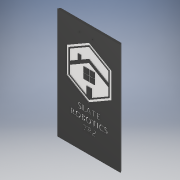
# Autodesk Inventor part: BA03
Saved by Autodesk Inventor 2017 (Build 210142000, 142)
## iProperties
Created: 2018-10-18
Part Number: BA03
Material: ABS Plastic
Document SubType Name: Modeling
Designer: Dell
Density: 1.06 g/cm^3
Appearance: Smooth - Black
Author: Dell
Autodesk Inventor part; units mm, degrees
ref_plane "YZ Plane" through (0, 0, 0) normal (1, 0, 0) x (0, 1, 0)
ref_plane "XZ Plane" through (0, 0, 0) normal (0, 1, 0) x (-1, 0, 0)
ref_plane "XY Plane" through (0, 0, 0) normal (0, 0, 1) x (1, 0, 0)
sketch "Sketch1" plane through (0, 0, 0) normal (0, 0, 1) x (1, 0, 0)
  line L0 (0, 0) -> (292.1, 0)
  line L1 (292.1, 0) -> (292.1, -533.4)
  line L2 (292.1, -533.4) -> (0, -533.4)
  line L3 (0, -533.4) -> (0, 0)
  dimension "d0" = 292.1
  dimension "d1" = 533.4
  constraints: 8 end point, 2 parallel, 1 horizontal, 1 perpendicular
  measures "d0" distance of L1.end L2.end
  measures "d1" distance of L0.end L1.end
extrude "Extrusion1" add sketch "Sketch1" along normal blind 10
sketch "Sketch2" plane through (0, 0, 0) normal (0, 1, 0) x (1, 0, 0)
  line L0 (292.1, -10) -> (0, -10) projected
  line L1 (0, -10) -> (-5.7735, -10)
  line L2 (-5.7735, -10) -> (0, 0)
  line L3 (0, 0) -> (0, -10) projected
  line L4 (0, 0) -> (0, -10) projected
  line L5 (0, -10) -> (0, 0)
  line L6 (292.1, -10) -> (297.8735, -10)
  line L7 (292.1, 0) -> (292.1, -10) projected
  line L8 (297.8735, -10) -> (292.1, 0)
  line L9 (292.1, 0) -> (292.1, -10)
  dimension "d4" = 30
  dimension "d5" = 60
  constraints: 12 end point, 2 collinear, 2 horizontal
  measures "d4" angle of L3 L2
  measures "d5" angle of L6 L8
extrude "Extrusion2" add sketch "Sketch2" against normal blind 533.4
sketch "Sketch5" plane through (0, 0, 10) normal (0, 0, 1) x (1, 0, 0)
  circle A0 centre (101, -44.45) radius 2.3812
  circle A1 centre (164.5, -44.45) radius 2.3813
  line L0 (-5.7735, 0) -> (297.8735, 0) projected
  line L1 (-5.7735, 0) -> (-5.7735, -533.4) projected
  line L2 (0, -533.4) -> (0, 0) projected
  dimension "d18" = 4.7625
  dimension "d19" = 63.5
  dimension "d20" = 4.7625
  dimension "d21" = 44.45
  dimension "d23" = 101
  constraints: 2 centre point, 1 horizontal alignment
  measures "d18" diameter of A0
  measures "d19" distance of A0.centre A1.centre
  measures "d20" diameter of A1
  measures "d21" distance from line of L0 A0.centre
  measures "d23" distance from line of A0.centre L2
extrude "Extrusion4" cut sketch "Sketch5" against normal through all
sketch "Sketch6" plane through (0, 0, 10) normal (0, 0, 1) x (1, 0, 0)
  line L0 (21.05, -316.7) -> (271.05, -316.7) construction
  line L1 (271.05, -316.7) -> (271.05, -466.7) construction
  line L2 (271.05, -466.7) -> (21.05, -466.7) construction
  line L3 (21.05, -466.7) -> (21.05, -316.7) construction
  line L4 (21.05, -66.7) -> (271.05, -66.7) construction
  line L5 (271.05, -66.7) -> (271.05, -316.7) construction
  line L6 (271.05, -316.7) -> (21.05, -316.7) construction
  line L7 (21.05, -316.7) -> (21.05, -66.7) construction
  line L8 (271.05, -466.7) -> (271.05, -66.7) construction
  line L9 (146.05, -66.7) -> (254.3032, -129.2)
  line L10 (254.3032, -129.2) -> (254.3032, -254.2)
  line L11 (254.3032, -254.2) -> (146.05, -316.7)
  line L12 (146.05, -316.7) -> (37.7968, -254.2)
  line L13 (37.7968, -254.2) -> (37.7968, -129.2)
  line L14 (37.7968, -129.2) -> (146.05, -66.7)
  line L15 (146.05, -78.4779) -> (244.1032, -135.089)
  line L16 (244.1032, -135.089) -> (244.1032, -248.311)
  line L17 (244.1032, -248.311) -> (146.05, -304.9221)
  line L18 (146.05, -304.9221) -> (47.9968, -248.311)
  line L19 (47.9968, -248.311) -> (47.9968, -135.089)
  line L20 (47.9968, -135.089) -> (146.05, -78.4779)
  line L21 (146.05, -83.3854) -> (239.8532, -137.5427) construction
  line L22 (239.8532, -137.5427) -> (239.8532, -245.8573) construction
  line L23 (239.8532, -245.8573) -> (146.05, -300.0146) construction
  line L24 (146.05, -300.0146) -> (52.2468, -245.8573) construction
  line L25 (52.2468, -245.8573) -> (52.2468, -137.5427) construction
  line L26 (52.2468, -137.5427) -> (146.05, -83.3854) construction
  line L27 (52.2468, -190.0427) -> (92.2468, -166.9487)
  line L28 (92.2468, -166.9487) -> (92.2468, -138.4487)
  line L29 (92.2468, -138.4487) -> (106.2468, -138.4487)
  line L30 (106.2468, -138.4487) -> (106.2468, -158.8658)
  line L31 (106.2468, -158.8658) -> (146.05, -135.8854)
  line L32 (146.05, -135.8854) -> (239.8532, -190.0427)
  line L33 (239.8532, -190.0427) -> (239.8532, -137.5427)
  line L34 (239.8532, -137.5427) -> (146.05, -83.3854)
  line L35 (146.05, -83.3854) -> (52.2468, -137.5427)
  line L36 (52.2468, -190.0427) -> (52.2468, -137.5427)
  line L37 (52.2468, -245.8573) -> (134.05, -293.0864)
  line L38 (134.05, -293.0864) -> (134.05, -253.0146)
  line L39 (134.05, -253.0146) -> (158.05, -253.0146)
  line L40 (158.05, -253.0146) -> (158.05, -293.0864)
  line L41 (158.05, -293.0864) -> (239.8532, -245.8573)
  line L42 (239.8532, -245.8573) -> (239.8532, -205.0427)
  line L43 (239.8532, -205.0427) -> (146.05, -150.8854)
  line L44 (146.05, -150.8854) -> (52.2468, -205.0427)
  line L45 (52.2468, -205.0427) -> (52.2468, -245.8573)
  line L46 (119.8, -179.0146) -> (172.3, -179.0146) construction
  line L47 (172.3, -179.0146) -> (172.3, -230.0146) construction
  line L48 (172.3, -230.0146) -> (119.8, -230.0146) construction
  line L49 (119.8, -230.0146) -> (119.8, -179.0146) construction
  line L50 (119.8, -230.0146) -> (143.8, -230.0146)
  line L51 (143.8, -230.0146) -> (143.8, -206.0146)
  line L52 (143.8, -206.0146) -> (119.8, -206.0146)
  line L53 (119.8, -206.0146) -> (119.8, -230.0146)
  line L54 (119.8, -179.0146) -> (143.8, -179.0146)
  line L55 (143.8, -179.0146) -> (143.8, -203.0146)
  line L56 (143.8, -203.0146) -> (119.8, -203.0146)
  line L57 (119.8, -203.0146) -> (119.8, -179.0146)
  line L58 (172.3, -179.0146) -> (148.3, -179.0146)
  line L59 (148.3, -179.0146) -> (148.3, -203.0146)
  line L60 (148.3, -203.0146) -> (172.3, -203.0146)
  line L61 (172.3, -203.0146) -> (172.3, -179.0146)
  line L62 (172.3, -230.0146) -> (148.3, -230.0146)
  line L63 (148.3, -230.0146) -> (148.3, -206.0146)
  line L64 (148.3, -206.0146) -> (172.3, -206.0146)
  line L65 (172.3, -206.0146) -> (172.3, -230.0146)
  line L66 (-5.7735, 0) -> (297.8735, 0) projected
  line L67 (-5.7735, 0) -> (-5.7735, -533.4) projected
  line L68 (92.7983, -364.3042) -> (92.7983, -360.0196)
  spline S0 degree 2 poles (92.7983, -360.0196) (95.7248, -361.2437) (98.6131, -361.7219) (99.8182, -361.7219) knots 0 0 0 1 2 2 2
  spline S1 degree 2 poles (99.8182, -361.7219) (101.9987, -361.7219) (104.1602, -359.7709) (104.1602, -358.3937) knots 0 0 0 1 2 2 2
  spline S2 degree 2 poles (104.1602, -358.3937) (104.1602, -357.3417) (103.5672, -356.5) knots 0 0 0 1 1 1
  spline S3 degree 2 poles (103.5672, -356.5) (102.9551, -355.6776) (100.6024, -354.3577) knots 0 0 0 1 1 1
  line L69 (100.6024, -354.3577) -> (98.9192, -353.4205)
  spline S4 degree 2 poles (98.9192, -353.4205) (95.304, -351.4121) (94.0416, -349.7097) knots 0 0 0 1 1 1
  spline S5 degree 2 poles (94.0416, -349.7097) (92.7409, -348.0073) (92.7409, -345.7694) knots 0 0 0 1 1 1
  spline S6 degree 2 poles (92.7409, -345.7694) (92.7409, -342.9385) (97.0638, -338.9216) (101.0997, -338.9216) knots 0 0 0 1 2 2 2
  spline S7 degree 2 poles (101.0997, -338.9216) (104.1219, -338.9216) (107.9092, -339.7824) knots 0 0 0 1 1 1
  line L70 (107.9092, -339.7824) -> (107.9092, -343.7801)
  spline S8 degree 2 poles (107.9092, -343.7801) (104.0263, -342.3455) (101.7501, -342.3455) knots 0 0 0 1 1 1
  spline S9 degree 2 poles (101.7501, -342.3455) (99.8564, -342.3455) (97.8863, -343.9905) (97.8863, -345.1382) knots 0 0 0 1 2 2 2
  spline S10 degree 2 poles (97.8863, -345.1382) (97.8863, -346.018) (98.4984, -346.764) knots 0 0 0 1 1 1
  spline S11 degree 2 poles (98.4984, -346.764) (99.0722, -347.5291) (101.4249, -348.8489) knots 0 0 0 1 1 1
  line L71 (101.4249, -348.8489) -> (103.2229, -349.8436)
  spline S12 degree 2 poles (103.2229, -349.8436) (107.3736, -352.158) (108.5022, -353.8604) knots 0 0 0 1 1 1
  spline S13 degree 2 poles (108.5022, -353.8604) (109.6307, -355.5819) (109.6307, -357.7242) knots 0 0 0 1 1 1
  spline S14 degree 2 poles (109.6307, -357.7242) (109.6307, -360.8038) (104.9444, -365.1458) (99.8373, -365.1458) knots 0 0 0 1 2 2 2
  spline S15 degree 2 poles (99.8373, -365.1458) (96.8151, -365.1458) (92.7983, -364.3042) knots 0 0 0 1 1 1
  line L72 (113.9536, -364.5337) -> (113.9536, -339.5337)
  line L73 (113.9536, -339.5337) -> (119.1564, -339.5337)
  line L74 (119.1564, -339.5337) -> (119.1564, -360.9951)
  line L75 (119.1564, -360.9951) -> (130.3078, -360.9951)
  line L76 (130.3078, -360.9951) -> (130.3078, -364.5337)
  line L77 (130.3078, -364.5337) -> (113.9536, -364.5337)
  line L78 (131.3216, -364.5337) -> (141.0194, -339.5337)
  line L79 (141.0194, -339.5337) -> (146.2413, -339.5337)
  line L80 (146.2413, -339.5337) -> (155.9773, -364.5337)
  line L81 (155.9773, -364.5337) -> (150.6407, -364.5337)
  line L82 (150.6407, -364.5337) -> (148.0393, -357.8581)
  line L83 (148.0393, -357.8581) -> (137.7103, -357.8581)
  line L84 (137.7103, -357.8581) -> (135.1089, -364.5337)
  line L85 (135.1089, -364.5337) -> (131.3216, -364.5337)
  line L86 (138.9919, -354.5299) -> (146.7386, -354.5299)
  line L87 (146.7386, -354.5299) -> (142.8748, -344.5643)
  line L88 (142.8748, -344.5643) -> (138.9919, -354.5299)
  line L89 (165.7325, -364.5337) -> (165.7325, -342.9767)
  line L90 (165.7325, -342.9767) -> (156.7807, -342.9767)
  line L91 (156.7807, -342.9767) -> (156.7807, -339.5337)
  line L92 (156.7807, -339.5337) -> (179.887, -339.5337)
  line L93 (179.887, -339.5337) -> (179.887, -342.9767)
  line L94 (179.887, -342.9767) -> (170.9352, -342.9767)
  line L95 (170.9352, -342.9767) -> (170.9352, -364.5337)
  line L96 (170.9352, -364.5337) -> (165.7325, -364.5337)
  line L97 (183.3683, -364.5337) -> (183.3683, -339.5337)
  line L98 (183.3683, -339.5337) -> (199.3782, -339.5337)
  line L99 (199.3782, -339.5337) -> (199.3782, -342.9767)
  line L100 (199.3782, -342.9767) -> (188.571, -342.9767)
  line L101 (188.571, -342.9767) -> (188.571, -349.9392)
  line L102 (188.571, -349.9392) -> (197.5037, -349.9392)
  line L103 (197.5037, -349.9392) -> (197.5037, -353.3822)
  line L104 (197.5037, -353.3822) -> (188.571, -353.3822)
  line L105 (188.571, -353.3822) -> (188.571, -360.9951)
  line L106 (188.571, -360.9951) -> (200.1816, -360.9951)
  line L107 (200.1816, -360.9951) -> (200.1816, -364.5337)
  line L108 (200.1816, -364.5337) -> (183.3683, -364.5337)
  line L109 (58.0336, -404.4902) -> (58.0336, -379.4902)
  line L110 (58.0336, -379.4902) -> (67.387, -379.4902)
  spline S16 degree 2 poles (67.387, -379.4902) (70.2562, -379.4902) (73.2593, -380.9248) (74.9999, -383.8514) (74.9999, -385.6876) knots 0 0 0 1 2 3 3 3
  spline S17 degree 2 poles (74.9999, -385.6876) (74.9999, -387.8873) (72.475, -391.7894) (70.1606, -392.8223) knots 0 0 0 1 2 2 2
  line L111 (70.1606, -392.8223) -> (78.3281, -404.4902)
  line L112 (78.3281, -404.4902) -> (71.9968, -404.4902)
  line L113 (71.9968, -404.4902) -> (65.7803, -394.276)
  line L114 (65.7803, -394.276) -> (62.9303, -394.276)
  line L115 (62.9303, -394.276) -> (62.9303, -404.4902)
  line L116 (62.9303, -404.4902) -> (58.0336, -404.4902)
  line L117 (62.9303, -390.8521) -> (64.1162, -390.8521)
  spline S18 degree 2 poles (64.1162, -390.8521) (67.3297, -390.8521) (69.7971, -388.0403) (69.7971, -386.2615) knots 0 0 0 1 2 2 2
  spline S19 degree 2 poles (69.7971, -386.2615) (69.7971, -384.7312) (67.8078, -382.9141) (64.7474, -382.9141) knots 0 0 0 1 2 2 2
  line L118 (64.7474, -382.9141) -> (62.9303, -382.9141)
  line L119 (62.9303, -382.9141) -> (62.9303, -390.8521)
  spline S20 degree 2 poles (93.0183, -405.1023) (89.1162, -405.1023) (83.3396, -401.8697) (80.3365, -395.8253) (80.3365, -391.9807) knots 0 0 0 1 2 3 3 3
  spline S21 degree 2 poles (80.3365, -391.9807) (80.3365, -388.1742) (83.3396, -382.0916) (89.1544, -378.8781) (93.0183, -378.8781) knots 0 0 0 1 2 3 3 3
  spline S22 degree 2 poles (93.0183, -378.8781) (96.8629, -378.8781) (102.6778, -382.0916) (105.6808, -388.1742) (105.6808, -391.9807) knots 0 0 0 1 2 3 3 3
  spline S23 degree 2 poles (105.6808, -391.9807) (105.6808, -395.8253) (102.6778, -401.8697) (96.9203, -405.1023) (93.0183, -405.1023) knots 0 0 0 1 2 3 3 3
  spline S24 degree 2 poles (93.0183, -401.6784) (96.6334, -401.6784) (100.1529, -395.7871) (100.1529, -391.9807) knots 0 0 0 1 2 2 2
  spline S25 degree 2 poles (100.1529, -391.9807) (100.1529, -388.1551) (96.6143, -382.302) (93.0183, -382.302) knots 0 0 0 1 2 2 2
  spline S26 degree 2 poles (93.0183, -382.302) (89.4031, -382.302) (85.8645, -388.1551) (85.8645, -391.9807) knots 0 0 0 1 2 2 2
  spline S27 degree 2 poles (85.8645, -391.9807) (85.8645, -395.7871) (89.384, -401.6784) (93.0183, -401.6784) knots 0 0 0 1 2 2 2
  line L120 (110.348, -404.4902) -> (110.348, -379.4902)
  line L121 (110.348, -379.4902) -> (118.7834, -379.4902)
  spline S28 degree 2 poles (118.7834, -379.4902) (121.8438, -379.4902) (124.7704, -380.8674) (126.4345, -383.5453) (126.4345, -385.0564) knots 0 0 0 1 2 3 3 3
  spline S29 degree 2 poles (126.4345, -385.0564) (126.4345, -386.9309) (123.8331, -390.3739) (120.4666, -391.426) knots 0 0 0 1 2 2 2
  spline S30 degree 2 poles (120.4666, -391.426) (123.1445, -392.0954) (125.9754, -394.0465) (127.4482, -396.7626) (127.4482, -398.312) knots 0 0 0 1 2 3 3 3
  spline S31 degree 2 poles (127.4482, -398.312) (127.4482, -399.9952) (125.7267, -402.9217) (122.7046, -404.4902) (119.5676, -404.4902) knots 0 0 0 1 2 3 3 3
  line L122 (119.5676, -404.4902) -> (110.348, -404.4902)
  line L123 (115.3404, -400.9516) -> (116.335, -400.9516)
  spline S32 degree 2 poles (116.335, -400.9516) (119.0512, -400.9516) (121.0213, -400.2439) (122.016, -398.6563) (122.016, -397.6807) knots 0 0 0 1 2 3 3 3
  spline S33 degree 2 poles (122.016, -397.6807) (122.016, -395.8253) (118.7451, -393.2431) (116.2394, -393.2431) knots 0 0 0 1 2 2 2
  line L124 (116.2394, -393.2431) -> (115.3404, -393.2431)
  line L125 (115.3404, -393.2431) -> (115.3404, -400.9516)
  line L126 (115.3404, -389.8957) -> (116.4498, -389.8957)
  spline S34 degree 2 poles (116.4498, -389.8957) (118.8216, -389.8957) (121.1552, -387.543) (121.1552, -385.8598) knots 0 0 0 1 2 2 2
  spline S35 degree 2 poles (121.1552, -385.8598) (121.1552, -384.9608) (120.4666, -383.6409) (118.726, -382.9141) (116.2776, -382.9141) knots 0 0 0 1 2 3 3 3
  line L127 (116.2776, -382.9141) -> (115.3404, -382.9141)
  line L128 (115.3404, -382.9141) -> (115.3404, -389.8957)
  spline S36 degree 2 poles (143.2669, -405.1023) (139.3648, -405.1023) (133.5883, -401.8697) (130.5852, -395.8253) (130.5852, -391.9807) knots 0 0 0 1 2 3 3 3
  spline S37 degree 2 poles (130.5852, -391.9807) (130.5852, -388.1742) (133.5883, -382.0916) (139.4031, -378.8781) (143.2669, -378.8781) knots 0 0 0 1 2 3 3 3
  spline S38 degree 2 poles (143.2669, -378.8781) (147.1116, -378.8781) (152.9264, -382.0916) (155.9295, -388.1742) (155.9295, -391.9807) knots 0 0 0 1 2 3 3 3
  spline S39 degree 2 poles (155.9295, -391.9807) (155.9295, -395.8253) (152.9264, -401.8697) (147.169, -405.1023) (143.2669, -405.1023) knots 0 0 0 1 2 3 3 3
  spline S40 degree 2 poles (143.2669, -401.6784) (146.8821, -401.6784) (150.4016, -395.7871) (150.4016, -391.9807) knots 0 0 0 1 2 2 2
  spline S41 degree 2 poles (150.4016, -391.9807) (150.4016, -388.1551) (146.8629, -382.302) (143.2669, -382.302) knots 0 0 0 1 2 2 2
  spline S42 degree 2 poles (143.2669, -382.302) (139.6518, -382.302) (136.1131, -388.1551) (136.1131, -391.9807) knots 0 0 0 1 2 2 2
  spline S43 degree 2 poles (136.1131, -391.9807) (136.1131, -395.7871) (139.6326, -401.6784) (143.2669, -401.6784) knots 0 0 0 1 2 2 2
  line L129 (166.8132, -404.4902) -> (166.8132, -382.9332)
  line L130 (166.8132, -382.9332) -> (157.8614, -382.9332)
  line L131 (157.8614, -382.9332) -> (157.8614, -379.4902)
  line L132 (157.8614, -379.4902) -> (180.9678, -379.4902)
  line L133 (180.9678, -379.4902) -> (180.9678, -382.9332)
  line L134 (180.9678, -382.9332) -> (172.016, -382.9332)
  line L135 (172.016, -382.9332) -> (172.016, -404.4902)
  line L136 (172.016, -404.4902) -> (166.8132, -404.4902)
  line L137 (184.449, -404.4902) -> (184.449, -379.4902)
  line L138 (184.449, -379.4902) -> (189.6518, -379.4902)
  line L139 (189.6518, -379.4902) -> (189.6518, -404.4902)
  line L140 (189.6518, -404.4902) -> (184.449, -404.4902)
  spline S44 degree 2 poles (216.029, -403.4956) (214.384, -404.2224) (211.9547, -404.758) (208.8752, -405.1023) (207.3641, -405.1023) knots 0 0 0 1 2 3 3 3
  spline S45 degree 2 poles (207.3641, -405.1023) (200.8033, -405.1023) (194.3572, -397.719) (194.3572, -391.9807) knots 0 0 0 1 2 2 2
  spline S46 degree 2 poles (194.3572, -391.9807) (194.3572, -386.2423) (200.7841, -378.8781) (207.6893, -378.8781) knots 0 0 0 1 2 2 2
  spline S47 degree 2 poles (207.6893, -378.8781) (211.7635, -378.8781) (215.7994, -379.8345) knots 0 0 0 1 1 1
  line L141 (215.7994, -379.8345) -> (215.7994, -383.9087)
  spline S48 degree 2 poles (215.7994, -383.9087) (213.8484, -383.2393) (211.3809, -382.608) (209.1812, -382.302) (208.0718, -382.302) knots 0 0 0 1 2 3 3 3
  spline S49 degree 2 poles (208.0718, -382.302) (203.7681, -382.302) (199.8851, -387.8299) (199.8851, -391.9233) knots 0 0 0 1 2 2 2
  spline S50 degree 2 poles (199.8851, -391.9233) (199.8851, -396.2079) (204.2845, -401.5063) (208.6456, -401.5063) knots 0 0 0 1 2 2 2
  spline S51 degree 2 poles (208.6456, -401.5063) (212.2799, -401.5063) (216.029, -399.67) knots 0 0 0 1 1 1
  line L142 (216.029, -399.67) -> (216.029, -403.4956)
  line L143 (219.1468, -404.2607) -> (219.1468, -399.9761)
  spline S52 degree 2 poles (219.1468, -399.9761) (222.0733, -401.2002) (224.9616, -401.6784) (226.1667, -401.6784) knots 0 0 0 1 2 2 2
  spline S53 degree 2 poles (226.1667, -401.6784) (228.3473, -401.6784) (230.5087, -399.7274) (230.5087, -398.3502) knots 0 0 0 1 2 2 2
  spline S54 degree 2 poles (230.5087, -398.3502) (230.5087, -397.2982) (229.9157, -396.4566) knots 0 0 0 1 1 1
  spline S55 degree 2 poles (229.9157, -396.4566) (229.3036, -395.6341) (226.9509, -394.3142) knots 0 0 0 1 1 1
  line L144 (226.9509, -394.3142) -> (225.2677, -393.377)
  spline S56 degree 2 poles (225.2677, -393.377) (221.6525, -391.3686) (220.3901, -389.6662) knots 0 0 0 1 1 1
  spline S57 degree 2 poles (220.3901, -389.6662) (219.0894, -387.9638) (219.0894, -385.7259) knots 0 0 0 1 1 1
  spline S58 degree 2 poles (219.0894, -385.7259) (219.0894, -382.895) (223.4123, -378.8781) (227.4482, -378.8781) knots 0 0 0 1 2 2 2
  spline S59 degree 2 poles (227.4482, -378.8781) (230.4704, -378.8781) (234.2577, -379.7389) knots 0 0 0 1 1 1
  line L145 (234.2577, -379.7389) -> (234.2577, -383.7366)
  spline S60 degree 2 poles (234.2577, -383.7366) (230.3748, -382.302) (228.0986, -382.302) knots 0 0 0 1 1 1
  spline S61 degree 2 poles (228.0986, -382.302) (226.2049, -382.302) (224.2348, -383.947) (224.2348, -385.0947) knots 0 0 0 1 2 2 2
  spline S62 degree 2 poles (224.2348, -385.0947) (224.2348, -385.9745) (224.8469, -386.7205) knots 0 0 0 1 1 1
  spline S63 degree 2 poles (224.8469, -386.7205) (225.4207, -387.4856) (227.7734, -388.8054) knots 0 0 0 1 1 1
  line L146 (227.7734, -388.8054) -> (229.5714, -389.8001)
  spline S64 degree 2 poles (229.5714, -389.8001) (233.7222, -392.1146) (234.8507, -393.8169) knots 0 0 0 1 1 1
  spline S65 degree 2 poles (234.8507, -393.8169) (235.9792, -395.5384) (235.9792, -397.6807) knots 0 0 0 1 1 1
  spline S66 degree 2 poles (235.9792, -397.6807) (235.9792, -400.7603) (231.2929, -405.1023) (226.1858, -405.1023) knots 0 0 0 1 2 2 2
  spline S67 degree 2 poles (226.1858, -405.1023) (223.1636, -405.1023) (219.1468, -404.2607) knots 0 0 0 1 1 1
  line L147 (122.3962, -444.4784) -> (126.8577, -422.1322)
  line L148 (126.8577, -422.1322) -> (117.9731, -422.1322)
  line L149 (117.9731, -422.1322) -> (118.4923, -419.4784)
  line L150 (118.4923, -419.4784) -> (139.7808, -419.4784)
  line L151 (139.7808, -419.4784) -> (139.2423, -422.1322)
  line L152 (139.2423, -422.1322) -> (130.3769, -422.1322)
  line L153 (130.3769, -422.1322) -> (125.9346, -444.4784)
  line L154 (125.9346, -444.4784) -> (122.3962, -444.4784)
  line L155 (138.1846, -444.4784) -> (143.1654, -419.4784)
  line L156 (143.1654, -419.4784) -> (150.7038, -419.4784)
  spline S68 degree 2 poles (150.7038, -419.4784) (152.6846, -419.4784) (155.3962, -420.1515) (157.1846, -422.5745) (157.1846, -424.3245) knots 0 0 0 1 2 3 3 3
  spline S69 degree 2 poles (157.1846, -424.3245) (157.1846, -426.863) (153.5692, -431.363) (150.4923, -432.5361) knots 0 0 0 1 2 2 2
  line L157 (150.4923, -432.5361) -> (156.4346, -444.4784)
  line L158 (156.4346, -444.4784) -> (152.5115, -444.4784)
  line L159 (152.5115, -444.4784) -> (147.2615, -433.4207)
  line L160 (147.2615, -433.4207) -> (143.9154, -433.4207)
  line L161 (143.9154, -433.4207) -> (141.7231, -444.4784)
  line L162 (141.7231, -444.4784) -> (138.1846, -444.4784)
  line L163 (144.4346, -430.8053) -> (146.3962, -430.8053)
  spline S70 degree 2 poles (146.3962, -430.8053) (148.4923, -430.8053) (151.5885, -429.2284) (153.4154, -426.2284) (153.4154, -424.7284) knots 0 0 0 1 2 3 3 3
  spline S71 degree 2 poles (153.4154, -424.7284) (153.4154, -423.4399) (151.4538, -422.1322) (148.4154, -422.1322) knots 0 0 0 1 2 2 2
  line L164 (148.4154, -422.1322) -> (146.1654, -422.1322)
  line L165 (146.1654, -422.1322) -> (144.4346, -430.8053)
  line L166 (160.1269, -444.4784) -> (160.6654, -441.7861)
  spline S72 degree 2 poles (160.6654, -441.7861) (161.8, -439.7091) (165.0115, -436.4015) (167.3577, -434.5938) knots 0 0 0 1 2 2 2
  line L167 (167.3577, -434.5938) -> (169.4538, -432.9976)
  spline S73 degree 2 poles (169.4538, -432.9976) (172.4346, -430.7091) (174.0308, -428.7668) knots 0 0 0 1 1 1
  spline S74 degree 2 poles (174.0308, -428.7668) (174.8385, -427.7861) (175.6462, -425.8438) (175.6462, -424.8822) knots 0 0 0 1 2 2 2
  spline S75 degree 2 poles (175.6462, -424.8822) (175.6462, -423.3053) (173.4731, -421.363) (171.3385, -421.363) knots 0 0 0 1 2 2 2
  spline S76 degree 2 poles (171.3385, -421.363) (168.3385, -421.363) (164.7423, -423.4015) knots 0 0 0 1 1 1
  line L168 (164.7423, -423.4015) -> (165.3385, -420.4207)
  spline S77 degree 2 poles (165.3385, -420.4207) (165.9154, -420.2091) (166.1846, -420.0745) knots 0 0 0 1 1 1
  spline S78 degree 2 poles (166.1846, -420.0745) (169.4731, -418.863) (172.1846, -418.863) knots 0 0 0 1 1 1
  spline S79 degree 2 poles (172.1846, -418.863) (175.3769, -418.863) (179.1846, -421.6515) (179.1846, -424.4784) knots 0 0 0 1 2 2 2
  spline S80 degree 2 poles (179.1846, -424.4784) (179.1846, -425.9784) (178.6462, -427.3053) knots 0 0 0 1 1 1
  spline S81 degree 2 poles (178.6462, -427.3053) (177.8385, -429.3438) (174.8962, -432.1899) (172.1846, -434.1707) knots 0 0 0 1 2 2 2
  line L169 (172.1846, -434.1707) -> (170.0885, -435.6899)
  spline S82 degree 2 poles (170.0885, -435.6899) (168.2038, -437.0745) (166.8, -438.3822) (166.1462, -439.1707) knots 0 0 0 1 2 2 2
  spline S83 degree 2 poles (166.1462, -439.1707) (165.7615, -439.6707) (165.05, -440.6322) (164.6462, -441.5745) knots 0 0 0 1 2 2 2
  line L170 (164.6462, -441.5745) -> (175.6077, -441.5745)
  line L171 (175.6077, -441.5745) -> (175.0115, -444.4784)
  line L172 (175.0115, -444.4784) -> (160.1269, -444.4784)
  point P0 (0, 0)
  point P1 (146.05, -191.7)
  point P2 (146.05, -253.0146)
  point P3 (146.05, -179.0146)
  point P4 (271.05, -266.7)
  point P5 (-5.7735, -266.7)
  point P6 (146.05, 0)
  dimension "d27" = 250
  dimension "d28" = 10.2
  dimension "d29" = 4.25
  dimension "d30" = 52.5
  dimension "d31" = 40
  dimension "d32" = 14
  dimension "d33" = 28.5
  dimension "d34" = 15
  dimension "d35" = 24
  dimension "d36" = 47
  dimension "d37" = 23
  dimension "d38" = 51
  dimension "d39" = 52.5
  dimension "d40" = 24
  dimension "d41" = 24
  dimension "d42" = 24
  dimension "d43" = 24
  dimension "d44" = 24
  dimension "d45" = 24
  dimension "d46" = 24
  dimension "d47" = 24
  dimension "d66" = 150
  constraints: 116 end point, 15 parallel, 9 perpendicular, 9 point on line, 8 midpoint, 6 vertical alignment, 5 horizontal, 4 collinear, 2 coincident, 2 vertical, 1 horizontal alignment, 26 other
  measures "d27" distance of L7.end L5.start
  measures "d28" distance between parallel lines of L14 L20
  measures "d29" distance between parallel lines of L20 L26
  measures "d30" distance of L27.start L25.end
  measures "d31" distance between parallel lines of L25 L28
  measures "d32" distance of L28.end L29.end
  measures "d33" distance of L27.end L28.end
  measures "d34" distance of L32.start L43.end
  measures "d35" distance between parallel lines of L40 L38
  measures "d36" distance from line of L24.start L39
  measures "d37" distance between parallel lines of L39 L48
  measures "d38" distance of L50.start L54.start
  measures "d39" distance of L54.start L61.end
  measures "d40" distance of L52.end L52.start
  measures "d41" distance of L52.start L51.start
  measures "d42" distance of L55.end L57.start
  measures "d43" distance of L55.start L55.end
  measures "d44" distance of L61.start L59.end
  measures "d45" distance of L59.end L59.start
  measures "d46" distance of L64.start L64.end
  measures "d47" distance of L63.start L64.start
  measures "d66" distance between parallel lines of L2 L6
extrude "Extrusion5" cut sketch "Sketch6" against normal blind 2
body "Solid1"
